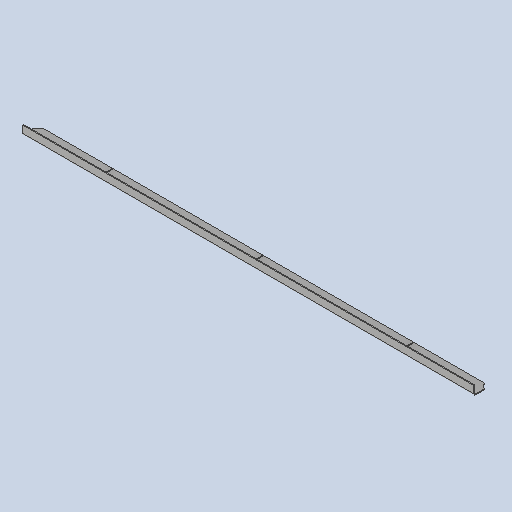
# Autodesk Inventor part: МОО 055 стрингер борт 51
Saved by Autodesk Inventor 2024.2 (Build 282272000, 272)
## iProperties
Created: 2024-04-28
Part Number: МОО 055 стрингер борт 51
Material: Generic
Document SubType Name: Sheet Metal
Designer: pokla
Density: 1 g/cm^3
Sheet Metal Rule: Default_mm
Appearance: Default
Author: admin
Autodesk Inventor part; units mm, degrees
ref_plane "YZ Plane" through (0, 0, 0) normal (1, 0, 0) x (0, 1, 0)
ref_plane "XZ Plane" through (0, 0, 0) normal (0, 1, 0) x (-1, 0, 0)
ref_plane "XY Plane" through (0, 0, 0) normal (0, 0, 1) x (1, 0, 0)
sketch "Sketch1" plane through (0, 0, 0) normal (0, 0, 1) x (1, 0, 0)
  line L0 (-750, 51.6997) -> (750, 51.6997)
  line L1 (750, 51.6997) -> (750, 0)
  line L2 (750, 0) -> (-750, 0)
  line L3 (-750, 0) -> (-750, 51.6997)
  point P0 (0, 0)
  point P1 (0, 0)
  dimension "d0" = 1500
  dimension "d1" = 51.6997
  measures "d0" distance of L1.end L2.end
  measures "d1" distance of L0.end L1.end
extrude "Plate1" add sketch "Sketch1" along normal blind 3
sketch "Sketch2" plane through (750, 3, 0) normal (0, -1, 0) x (1, 0, 0)
  line L0 (-1500, 0) -> (0, 0)
  line L1 (0, 0) -> (0, 30)
  line L2 (0, 30) -> (-1500, 30)
  line L3 (-1500, 30) -> (-1500, 0)
  constraints: 6 end point, 1 horizontal, 1 perpendicular, 1 vertical
edge flange "Flange1" height 30 angle 90 thickness 3 bend radius 3 thickness toward (0, -1, 0) relief straight relief width 3 relief depth 1.5 edges at (0, 0, 3) wall of the first edge with corners at (-750, 3, 0) (750, 3, 0) (750, 3, 30) (-750, 3, 30)
bend "Bend1"
corner "Corner1"
sketch "Sketch5" plane through (0, 0, 0) normal (0, 0, -1) x (-1, 0, 0)
  line L0 (750, 51.6997) -> (-750, 51.6997) projected
  line L1 (500, 51.6997) -> (500, 31)
  line L2 (500, 31) -> (503, 31)
  line L3 (503, 31) -> (503, 51.6997)
  line L4 (750, 0) -> (-750, 0) projected
  point P0 (0, 0)
  dimension "d18" = 3
  dimension "d19" = 247
  dimension "d20" = 31
  constraints: 6 end point, 2 perpendicular, 2 point on line, 1 vertical
  measures "d18" distance between parallel lines of L3 L1
  measures "d19" distance from line of L0.start L3
  measures "d20" distance between parallel lines of L4 L2
extrude "Extrusion1" cut sketch "Sketch5" against normal through all
pattern_linear "Rectangular Pattern1" count 3 spacing 500 along (1, 0, 0) of "Extrusion1"
sketch "Sketch6" plane through (0, 0, 0) normal (0, 0, -1) x (-1, 0, 0)
  line L0 (-750, 51.6997) -> (-750, 6) projected
  circle A0 centre (-750, 51.6997) radius 15
  line L1 (-750, 51.6997) -> (-500, 51.6997) projected
  point P0 (0, 0)
  point P1 (-735, 51.6997)
  point P2 (-750, 36.6997)
  dimension "d24" = 30
  constraints: 1 centre point
  measures "d24" diameter of A0
extrude "Extrusion2" cut sketch "Sketch6" against normal through all contours L1 A0 L0 picked at (-740.1254, 50.5871)
mirror "Mirror1" about plane through (0, 0, 0) normal (1, 0, 0) of "Extrusion2"
equation "\"d1\" = Стрингер_5"
equation "\"d18\" = Thickness"
equation "\"d2\" = Thickness"
equation "\"d3\" = BendReliefWidth"
equation "\"d4\" = BendReliefDepth"
equation "\"d5\" = MinimumRemnant"
equation "\"d6\" = TransitionRadius"
equation "\"d9\" = BendRadius"
equation "\"d10\" = CornerReliefSize"
equation "\"d11\" = GapSize"
equation "\"d12\" = JacobiRadiusSize"
equation "\"BendRadius\" = Thickness"
equation "\"BendReliefWidth\" = Thickness"
equation "\"BendReliefDepth\" = 0.5 * Thickness"
equation "\"CornerReliefSize\" = 4 * Thickness"
equation "\"MinimumRemnant\" = 2 * Thickness"
equation "\"TransitionRadius\" = BendRadius"
equation "\"JacobiRadiusSize\" = BendRadius"
equation "\"GapSize\" = Thickness"
equation "\"Стрингер_5\" = 51.699679"
equation "\"Thickness\" = 3"
body "Solid1"
